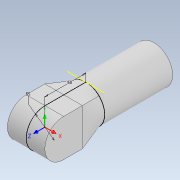
# Autodesk Inventor part: shank_2
Saved by Autodesk Inventor 2020 (Build 240168000, 168)
## iProperties
Created: 2021-01-30
Part Number: shank_2
Material: Generic
Document SubType Name: Modeling
Designer: DELL
Density: 1 g/cm^3
Appearance: Default
Author: DELL
Autodesk Inventor part; units mm, degrees
ref_plane "YZ Plane" through (0, 0, 0) normal (1, 0, 0) x (0, 1, 0)
ref_plane "XZ Plane" through (0, 0, 0) normal (0, 1, 0) x (-1, 0, 0)
ref_plane "UCS1: YZ Plane" through (0, 0, 0) normal (1, 0, 0) x (0, 1, 0)
sketch "Sketch6" plane through (0, 0, 0) normal (1, 0, 0) x (0, 1, 0)
  circle A0 centre (0, 0) radius 27.5
  line L0 (-27.5, 0) -> (-27.5, -60)
  line L1 (-27.5, -60) -> (27.5, -60)
  line L2 (27.5, -60) -> (27.5, 0)
  line L3 (0, 0) -> (0, -60) construction
  line L4 (-27.5, -27.5) -> (27.5, -27.5)
  dimension "d38" = 55
  dimension "d39" = 60
  constraints: 10 end point, 3 perpendicular, 2 point on circle, 2 point on line, 2 tangent, 2 vertical, 1 centre point, 1 coincident, 1 midpoint
  measures "d38" diameter of A0
  measures "d39" distance from line of L1 point (0, 0)
extrude "Extrusion8" add sketch "Sketch6" along normal mid plane 55 contours A0 | L2 L4 A0 | A0 L4 L0
ref_plane "Work Plane2" through (0, -27.5, -60) normal (0, 0, -1) x (0, 1, 0)
ref_plane "Work Plane1" through (0, 0, 27.5) normal (0, 0, 1) x (1, 0, 0)
sketch "Sketch3" plane through (0, -27.5, -60) normal (0, 0, -1) x (0, 1, 0)
  circle A0 centre (27.5, 0) radius 27.5
  line L0 (55, -27.5) -> (55, 27.5) projected
  constraints: 1 centre point, 1 coincident, 1 tangent
loft "Loft1" add profiles "Sketch3" separate body section 1 edges at (0, 27.5, -27.5) (27.5, 0, -27.5) (0, -27.5, -27.5) (-27.5, 0, -27.5)
extrude "Extrusion1" add sketch "Sketch3" along normal blind 100 bodies 2
sketch "Sketch5" plane through (0, 0, -160) normal (0, 0, -1) x (-1, 0, 0)
  circle A0 centre (0, 0) radius 12.5
  point P0 (0, 0)
  dimension "d35" = 25
  constraints: 1 centre point, 1 coincident
  measures "d35" diameter of A0
extrude "Extrusion7" cut sketch "Sketch5" against normal blind 60 bodies 2
body "Solid1"
body "Solid4"
